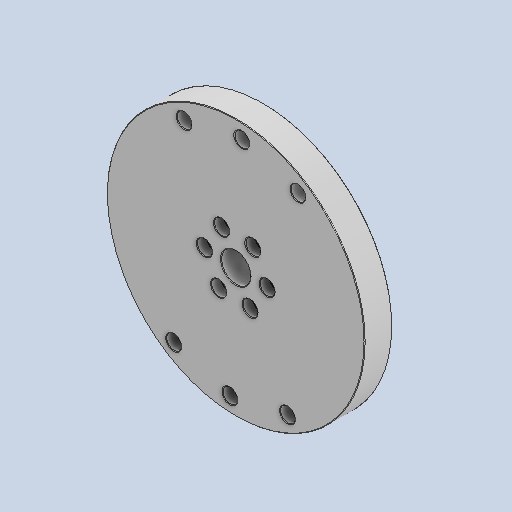
# Autodesk Inventor part: Góra
Saved by Autodesk Inventor 2023 (Build 270158000, 158)
## iProperties
Created: 2022-12-12
Part Number: Góra
Material: Generic
Document SubType Name: Modeling
Designer: komputer
Density: 1 g/cm^3
Appearance: Default
Author: komputer
Autodesk Inventor part; units mm, degrees
ref_plane "YZ Plane" through (0, 0, 0) normal (1, 0, 0) x (0, 1, 0)
ref_plane "XZ Plane" through (0, 0, 0) normal (0, 1, 0) x (-1, 0, 0)
ref_plane "XY Plane" through (0, 0, 0) normal (0, 0, 1) x (1, 0, 0)
sketch "Sketch1" plane through (0, 0, 0) normal (0, 0, 1) x (1, 0, 0)
  circle A0 centre (-9.0642, 40.3091) radius 2 projected
  circle A1 centre (-10.6114, 10.7871) radius 2 projected
  circle A2 centre (15.729, 24.2082) radius 2 projected
  circle A3 centre (6.4332, 9.8938) radius 2 projected
  circle A4 centre (-18.3601, 25.9947) radius 2 projected
  circle A5 centre (7.9804, 39.4158) radius 2 projected
  circle A6 centre (-1.3155, 25.1014) radius 9 projected
  circle A7 centre (-1.3155, 25.1014) radius 24.1359 projected
  circle A8 centre (-1.3155, 25.1014) radius 25 projected
  circle A9 centre (-9.0642, 40.3091) radius 3.5 projected
  circle A10 centre (-10.6114, 10.7871) radius 3.5 projected
  circle A11 centre (15.729, 24.2082) radius 3.5 projected
  circle A12 centre (6.4332, 9.8938) radius 3.5 projected
  circle A13 centre (-18.3601, 25.9947) radius 3.5 projected
  circle A14 centre (7.9804, 39.4158) radius 3.5 projected
  arc A15 (-0.8701, 59.0939) -> (-1.7609, 59.0939) centre (-1.3155, 25.1014) ccw projected
  arc A16 (1.7947, 58.9543) -> (-0.8701, 59.0939) centre (-1.3155, 25.1014) ccw projected
  arc A17 (2.6806, 58.8612) -> (1.7947, 58.9543) centre (-1.3155, 25.1014) ccw projected
  arc A18 (5.3163, 58.4437) -> (2.6806, 58.8612) centre (-1.3155, 25.1014) ccw projected
  arc A19 (6.1876, 58.2585) -> (5.3163, 58.4437) centre (-1.3155, 25.1014) ccw projected
  arc A20 (8.7652, 57.5678) -> (6.1876, 58.2585) centre (-1.3155, 25.1014) ccw projected
  arc A21 (9.6123, 57.2926) -> (8.7652, 57.5678) centre (-1.3155, 25.1014) ccw projected
  arc A22 (12.1036, 56.3363) -> (9.6123, 57.2926) centre (-1.3155, 25.1014) ccw projected
  arc A23 (12.9173, 55.974) -> (12.1036, 56.3363) centre (-1.3155, 25.1014) ccw projected
  arc A24 (15.295, 54.7625) -> (12.9173, 55.974) centre (-1.3155, 25.1014) ccw projected
  arc A25 (16.0664, 54.3171) -> (15.295, 54.7625) centre (-1.3155, 25.1014) ccw projected
  arc A26 (18.3044, 52.8637) -> (16.0664, 54.3171) centre (-1.3155, 25.1014) ccw projected
  arc A27 (19.0251, 52.3401) -> (18.3044, 52.8637) centre (-1.3155, 25.1014) ccw projected
  arc A28 (21.0989, 50.6608) -> (19.0251, 52.3401) centre (-1.3155, 25.1014) ccw projected
  arc A29 (21.7609, 50.0648) -> (21.0989, 50.6608) centre (-1.3155, 25.1014) ccw projected
  arc A30 (23.6478, 48.1778) -> (21.7609, 50.0648) centre (-1.3155, 25.1014) ccw projected
  arc A31 (24.2438, 47.5159) -> (23.6478, 48.1778) centre (-1.3155, 25.1014) ccw projected
  arc A32 (25.9232, 45.442) -> (24.2438, 47.5159) centre (-1.3155, 25.1014) ccw projected
  arc A33 (26.4468, 44.7214) -> (25.9232, 45.442) centre (-1.3155, 25.1014) ccw projected
  arc A34 (27.9002, 42.4834) -> (26.4468, 44.7214) centre (-1.3155, 25.1014) ccw projected
  arc A35 (28.3455, 41.712) -> (27.9002, 42.4834) centre (-1.3155, 25.1014) ccw projected
  arc A36 (29.557, 39.3343) -> (28.3455, 41.712) centre (-1.3155, 25.1014) ccw projected
  arc A37 (29.9193, 38.5206) -> (29.557, 39.3343) centre (-1.3155, 25.1014) ccw projected
  arc A38 (30.8756, 36.0293) -> (29.9193, 38.5206) centre (-1.3155, 25.1014) ccw projected
  arc A39 (31.1509, 35.1821) -> (30.8756, 36.0293) centre (-1.3155, 25.1014) ccw projected
  arc A40 (31.8416, 32.6045) -> (31.1509, 35.1821) centre (-1.3155, 25.1014) ccw projected
  arc A41 (32.0268, 31.7332) -> (31.8416, 32.6045) centre (-1.3155, 25.1014) ccw projected
  arc A42 (32.4442, 29.0976) -> (32.0268, 31.7332) centre (-1.3155, 25.1014) ccw projected
  arc A43 (32.5373, 28.2117) -> (32.4442, 29.0976) centre (-1.3155, 25.1014) ccw projected
  arc A44 (32.677, 25.5468) -> (32.5373, 28.2117) centre (-1.3155, 25.1014) ccw projected
  arc A45 (32.677, 24.6561) -> (32.677, 25.5468) centre (-1.3155, 25.1014) ccw projected
  arc A46 (32.5373, 21.9912) -> (32.677, 24.6561) centre (-1.3155, 25.1014) ccw projected
  arc A47 (32.4442, 21.1053) -> (32.5373, 21.9912) centre (-1.3155, 25.1014) ccw projected
  arc A48 (32.0268, 18.4697) -> (32.4442, 21.1053) centre (-1.3155, 25.1014) ccw projected
  arc A49 (31.8416, 17.5984) -> (32.0268, 18.4697) centre (-1.3155, 25.1014) ccw projected
  arc A50 (31.1509, 15.0208) -> (31.8416, 17.5984) centre (-1.3155, 25.1014) ccw projected
  arc A51 (30.8756, 14.1736) -> (31.1509, 15.0208) centre (-1.3155, 25.1014) ccw projected
  arc A52 (29.9193, 11.6823) -> (30.8756, 14.1736) centre (-1.3155, 25.1014) ccw projected
  arc A53 (29.557, 10.8686) -> (29.9193, 11.6823) centre (-1.3155, 25.1014) ccw projected
  arc A54 (28.3455, 8.4909) -> (29.557, 10.8686) centre (-1.3155, 25.1014) ccw projected
  arc A55 (27.9002, 7.7195) -> (28.3455, 8.4909) centre (-1.3155, 25.1014) ccw projected
  arc A56 (26.4468, 5.4815) -> (27.9002, 7.7195) centre (-1.3155, 25.1014) ccw projected
  arc A57 (25.9232, 4.7608) -> (26.4468, 5.4815) centre (-1.3155, 25.1014) ccw projected
  arc A58 (24.2438, 2.687) -> (25.9232, 4.7608) centre (-1.3155, 25.1014) ccw projected
  arc A59 (23.6478, 2.0251) -> (24.2438, 2.687) centre (-1.3155, 25.1014) ccw projected
  arc A60 (21.7609, 0.1381) -> (23.6478, 2.0251) centre (-1.3155, 25.1014) ccw projected
  arc A61 (21.0989, -0.4579) -> (21.7609, 0.1381) centre (-1.3155, 25.1014) ccw projected
  arc A62 (19.0251, -2.1373) -> (21.0989, -0.4579) centre (-1.3155, 25.1014) ccw projected
  arc A63 (18.3044, -2.6608) -> (19.0251, -2.1373) centre (-1.3155, 25.1014) ccw projected
  arc A64 (16.0664, -4.1142) -> (18.3044, -2.6608) centre (-1.3155, 25.1014) ccw projected
  arc A65 (15.295, -4.5596) -> (16.0664, -4.1142) centre (-1.3155, 25.1014) ccw projected
  arc A66 (12.9173, -5.7711) -> (15.295, -4.5596) centre (-1.3155, 25.1014) ccw projected
  arc A67 (12.1036, -6.1334) -> (12.9173, -5.7711) centre (-1.3155, 25.1014) ccw projected
  arc A68 (9.6123, -7.0897) -> (12.1036, -6.1334) centre (-1.3155, 25.1014) ccw projected
  arc A69 (8.7652, -7.365) -> (9.6123, -7.0897) centre (-1.3155, 25.1014) ccw projected
  arc A70 (6.1876, -8.0556) -> (8.7652, -7.365) centre (-1.3155, 25.1014) ccw projected
  arc A71 (5.3163, -8.2408) -> (6.1876, -8.0556) centre (-1.3155, 25.1014) ccw projected
  arc A72 (2.6806, -8.6583) -> (5.3163, -8.2408) centre (-1.3155, 25.1014) ccw projected
  arc A73 (1.7947, -8.7514) -> (2.6806, -8.6583) centre (-1.3155, 25.1014) ccw projected
  arc A74 (-0.8701, -8.891) -> (1.7947, -8.7514) centre (-1.3155, 25.1014) ccw projected
  arc A75 (-1.7609, -8.891) -> (-0.8701, -8.891) centre (-1.3155, 25.1014) ccw projected
  arc A76 (-4.4258, -8.7514) -> (-1.7609, -8.891) centre (-1.3155, 25.1014) ccw projected
  arc A77 (-5.3116, -8.6583) -> (-4.4258, -8.7514) centre (-1.3155, 25.1014) ccw projected
  arc A78 (-7.9473, -8.2408) -> (-5.3116, -8.6583) centre (-1.3155, 25.1014) ccw projected
  arc A79 (-8.8186, -8.0556) -> (-7.9473, -8.2408) centre (-1.3155, 25.1014) ccw projected
  arc A80 (-11.3962, -7.365) -> (-8.8186, -8.0556) centre (-1.3155, 25.1014) ccw projected
  arc A81 (-12.2433, -7.0897) -> (-11.3962, -7.365) centre (-1.3155, 25.1014) ccw projected
  arc A82 (-14.7346, -6.1334) -> (-12.2433, -7.0897) centre (-1.3155, 25.1014) ccw projected
  arc A83 (-15.5484, -5.7711) -> (-14.7346, -6.1334) centre (-1.3155, 25.1014) ccw projected
  arc A84 (-17.926, -4.5596) -> (-15.5484, -5.7711) centre (-1.3155, 25.1014) ccw projected
  arc A85 (-18.6975, -4.1142) -> (-17.926, -4.5596) centre (-1.3155, 25.1014) ccw projected
  arc A86 (-20.9355, -2.6608) -> (-18.6975, -4.1142) centre (-1.3155, 25.1014) ccw projected
  arc A87 (-21.6561, -2.1373) -> (-20.9355, -2.6608) centre (-1.3155, 25.1014) ccw projected
  arc A88 (-23.7299, -0.4579) -> (-21.6561, -2.1373) centre (-1.3155, 25.1014) ccw projected
  arc A89 (-24.3919, 0.1381) -> (-23.7299, -0.4579) centre (-1.3155, 25.1014) ccw projected
  arc A90 (-26.2788, 2.0251) -> (-24.3919, 0.1381) centre (-1.3155, 25.1014) ccw projected
  arc A91 (-26.8749, 2.687) -> (-26.2788, 2.0251) centre (-1.3155, 25.1014) ccw projected
  arc A92 (-28.5542, 4.7608) -> (-26.8749, 2.687) centre (-1.3155, 25.1014) ccw projected
  arc A93 (-29.0778, 5.4815) -> (-28.5542, 4.7608) centre (-1.3155, 25.1014) ccw projected
  arc A94 (-30.5312, 7.7195) -> (-29.0778, 5.4815) centre (-1.3155, 25.1014) ccw projected
  arc A95 (-30.9766, 8.4909) -> (-30.5312, 7.7195) centre (-1.3155, 25.1014) ccw projected
  arc A96 (-32.188, 10.8686) -> (-30.9766, 8.4909) centre (-1.3155, 25.1014) ccw projected
  arc A97 (-32.5503, 11.6823) -> (-32.188, 10.8686) centre (-1.3155, 25.1014) ccw projected
  arc A98 (-33.5067, 14.1736) -> (-32.5503, 11.6823) centre (-1.3155, 25.1014) ccw projected
  arc A99 (-33.7819, 15.0208) -> (-33.5067, 14.1736) centre (-1.3155, 25.1014) ccw projected
  arc A100 (-34.4726, 17.5984) -> (-33.7819, 15.0208) centre (-1.3155, 25.1014) ccw projected
  arc A101 (-34.6578, 18.4697) -> (-34.4726, 17.5984) centre (-1.3155, 25.1014) ccw projected
  arc A102 (-35.0752, 21.1053) -> (-34.6578, 18.4697) centre (-1.3155, 25.1014) ccw projected
  arc A103 (-35.1683, 21.9912) -> (-35.0752, 21.1053) centre (-1.3155, 25.1014) ccw projected
  arc A104 (-35.308, 24.6561) -> (-35.1683, 21.9912) centre (-1.3155, 25.1014) ccw projected
  arc A105 (-35.308, 25.5468) -> (-35.308, 24.6561) centre (-1.3155, 25.1014) ccw projected
  arc A106 (-35.1683, 28.2117) -> (-35.308, 25.5468) centre (-1.3155, 25.1014) ccw projected
  arc A107 (-35.0752, 29.0976) -> (-35.1683, 28.2117) centre (-1.3155, 25.1014) ccw projected
  arc A108 (-34.6578, 31.7332) -> (-35.0752, 29.0976) centre (-1.3155, 25.1014) ccw projected
  arc A109 (-34.4726, 32.6045) -> (-34.6578, 31.7332) centre (-1.3155, 25.1014) ccw projected
  arc A110 (-33.7819, 35.1821) -> (-34.4726, 32.6045) centre (-1.3155, 25.1014) ccw projected
  arc A111 (-33.5067, 36.0293) -> (-33.7819, 35.1821) centre (-1.3155, 25.1014) ccw projected
  arc A112 (-32.5503, 38.5206) -> (-33.5067, 36.0293) centre (-1.3155, 25.1014) ccw projected
  arc A113 (-32.188, 39.3343) -> (-32.5503, 38.5206) centre (-1.3155, 25.1014) ccw projected
  arc A114 (-30.9766, 41.712) -> (-32.188, 39.3343) centre (-1.3155, 25.1014) ccw projected
  arc A115 (-30.5312, 42.4834) -> (-30.9766, 41.712) centre (-1.3155, 25.1014) ccw projected
  arc A116 (-29.0778, 44.7214) -> (-30.5312, 42.4834) centre (-1.3155, 25.1014) ccw projected
  arc A117 (-28.5542, 45.442) -> (-29.0778, 44.7214) centre (-1.3155, 25.1014) ccw projected
  arc A118 (-26.8749, 47.5159) -> (-28.5542, 45.442) centre (-1.3155, 25.1014) ccw projected
  arc A119 (-26.2788, 48.1778) -> (-26.8749, 47.5159) centre (-1.3155, 25.1014) ccw projected
  arc A120 (-24.3919, 50.0648) -> (-26.2788, 48.1778) centre (-1.3155, 25.1014) ccw projected
  arc A121 (-23.7299, 50.6608) -> (-24.3919, 50.0648) centre (-1.3155, 25.1014) ccw projected
  arc A122 (-21.6561, 52.3401) -> (-23.7299, 50.6608) centre (-1.3155, 25.1014) ccw projected
  arc A123 (-20.9355, 52.8637) -> (-21.6561, 52.3401) centre (-1.3155, 25.1014) ccw projected
  arc A124 (-18.6975, 54.3171) -> (-20.9355, 52.8637) centre (-1.3155, 25.1014) ccw projected
  arc A125 (-17.926, 54.7625) -> (-18.6975, 54.3171) centre (-1.3155, 25.1014) ccw projected
  arc A126 (-15.5484, 55.974) -> (-17.926, 54.7625) centre (-1.3155, 25.1014) ccw projected
  arc A127 (-14.7346, 56.3363) -> (-15.5484, 55.974) centre (-1.3155, 25.1014) ccw projected
  arc A128 (-12.2433, 57.2926) -> (-14.7346, 56.3363) centre (-1.3155, 25.1014) ccw projected
  arc A129 (-11.3962, 57.5678) -> (-12.2433, 57.2926) centre (-1.3155, 25.1014) ccw projected
  arc A130 (-8.8186, 58.2585) -> (-11.3962, 57.5678) centre (-1.3155, 25.1014) ccw projected
  arc A131 (-7.9473, 58.4437) -> (-8.8186, 58.2585) centre (-1.3155, 25.1014) ccw projected
  arc A132 (-5.3116, 58.8612) -> (-7.9473, 58.4437) centre (-1.3155, 25.1014) ccw projected
  arc A133 (-4.4258, 58.9543) -> (-5.3116, 58.8612) centre (-1.3155, 25.1014) ccw projected
  arc A134 (-1.7609, 59.0939) -> (-4.4258, 58.9543) centre (-1.3155, 25.1014) ccw projected
  circle A135 centre (-1.3155, 25.1014) radius 9 projected
  circle A136 centre (-1.3155, 25.1014) radius 8 projected
  point P0 (0, 0)
extrude "Extrusion1" add sketch "Sketch1" along normal blind 37 contours A6 | A7 | A9 | A10 | A11 | A12 | A13 | A14
sketch "Sketch2" plane through (-1.3155, 25.1014, 37) normal (0, 0, 1) x (1, 0, 0)
  circle A0 centre (0, 0) radius 43.6804 projected
  circle A1 centre (0, 0) radius 8 projected
  circle A2 centre (0, 0) radius 50
  circle A3 centre (0, 0) radius 24.1359 projected
  circle A4 centre (9.2959, 14.3144) radius 2 projected
  circle A5 centre (-17.0446, 0.8933) radius 2 projected
  circle A6 centre (7.7487, -15.2076) radius 2 projected
  circle A7 centre (17.0446, -0.8933) radius 2 projected
  circle A8 centre (-9.2959, -14.3144) radius 2 projected
  circle A9 centre (-7.7487, 15.2076) radius 2 projected
  circle A10 centre (0, 0) radius 8 projected
  point P0 (1.3155, -25.1014)
  dimension "d2" = 100
  constraints: 1 centre point, 1 coincident
  measures "d2" diameter of A2
extrude "Extrusion2" add sketch "Sketch2" against normal blind 10 contours A0 | A2
sketch "Sketch3" plane through (-1.3155, 25.1014, 37) normal (0, 0, 1) x (1, 0, 0)
  circle A0 centre (0, 0) radius 55
  circle A1 centre (0, 0) radius 50 projected
  circle A2 centre (9.2959, 14.3144) radius 2 projected
  circle A3 centre (-17.0446, 0.8933) radius 2 projected
  circle A4 centre (7.7487, -15.2076) radius 2 projected
  circle A5 centre (17.0446, -0.8933) radius 2 projected
  circle A6 centre (-9.2959, -14.3144) radius 2 projected
  circle A7 centre (-7.7487, 15.2076) radius 2 projected
  circle A8 centre (0, 0) radius 8 projected
  point P0 (1.3155, -25.1014)
  constraints: 1 centre point, 2 other
ref_plane "Work Plane1" through (-65.2569, -38.84, 26) normal (0, 0, 1) x (0.9839108, 0.1786605, 0)
extrude "Extrusion3" add sketch "Sketch3" against normal blind 10 contours A0
sketch "Sketch4" plane through (-1.3155, 25.1014, 37) normal (0, 0, 1) x (1, 0, 0)
  circle A0 centre (0, 0) radius 55 projected
  circle A1 centre (9.2959, 14.3144) radius 2 projected
  circle A2 centre (-17.0446, 0.8933) radius 2 projected
  circle A3 centre (7.7487, -15.2076) radius 2 projected
  circle A4 centre (17.0446, -0.8933) radius 2 projected
  circle A5 centre (-9.2959, -14.3144) radius 2 projected
  circle A6 centre (-7.7487, 15.2076) radius 2 projected
  circle A7 centre (0, 0) radius 8 projected
  line L0 (-9.2959, -14.3144) -> (-9.2959, -10.8144)
  line L1 (-9.2959, -10.8144) -> (-9.2959, -17.4144)
  line L2 (-11.0857, -17.4144) -> (-12.8754, -14.3144)
  line L3 (-12.8754, -14.3144) -> (-11.0857, -11.2144)
  line L4 (-11.0857, -11.2144) -> (-7.5061, -11.2144)
  line L5 (-7.5061, -11.2144) -> (-5.7163, -14.3144)
  line L6 (-5.7163, -14.3144) -> (-7.5061, -17.4144)
  line L7 (-7.5061, -17.4144) -> (-11.0857, -17.4144)
  line L8 (9.5385, -12.1076) -> (11.3283, -15.2076)
  line L9 (9.5385, -18.3076) -> (5.9589, -18.3076)
  line L10 (5.9589, -18.3076) -> (4.1691, -15.2076)
  line L11 (11.3283, -15.2076) -> (9.5385, -18.3076)
  line L12 (4.1691, -15.2076) -> (5.9589, -12.1076)
  line L13 (5.9589, -12.1076) -> (9.5385, -12.1076)
  line L14 (15.2548, 2.2067) -> (18.8343, 2.2067)
  line L15 (20.6241, -0.8933) -> (18.8343, -3.9933)
  line L16 (18.8343, -3.9933) -> (15.2548, -3.9933)
  line L17 (18.8343, 2.2067) -> (20.6241, -0.8933)
  line L18 (15.2548, -3.9933) -> (13.465, -0.8933)
  line L19 (13.465, -0.8933) -> (15.2548, 2.2067)
  line L20 (5.7163, 14.3144) -> (7.5061, 17.4144)
  line L21 (11.0857, 17.4144) -> (12.8754, 14.3144)
  line L22 (12.8754, 14.3144) -> (11.0857, 11.2144)
  line L23 (7.5061, 17.4144) -> (11.0857, 17.4144)
  line L24 (11.0857, 11.2144) -> (7.5061, 11.2144)
  line L25 (7.5061, 11.2144) -> (5.7163, 14.3144)
  line L26 (-9.5385, 12.1076) -> (-11.3283, 15.2076)
  line L27 (-9.5385, 18.3076) -> (-5.9589, 18.3076)
  line L28 (-5.9589, 18.3076) -> (-4.1691, 15.2076)
  line L29 (-11.3283, 15.2076) -> (-9.5385, 18.3076)
  line L30 (-4.1691, 15.2076) -> (-5.9589, 12.1076)
  line L31 (-5.9589, 12.1076) -> (-9.5385, 12.1076)
  line L32 (-15.2548, -2.2067) -> (-18.8343, -2.2067)
  line L33 (-20.6241, 0.8933) -> (-18.8343, 3.9933)
  line L34 (-18.8343, 3.9933) -> (-15.2548, 3.9933)
  line L35 (-18.8343, -2.2067) -> (-20.6241, 0.8933)
  line L36 (-15.2548, 3.9933) -> (-13.465, 0.8933)
  line L37 (-13.465, 0.8933) -> (-15.2548, -2.2067)
  point P0 (1.3155, -25.1014)
  point P1 (10.4334, -16.7576)
  point P2 (7.7487, -15.2076)
  point P3 (4.7176, -13.4576)
  point P4 (19.7292, 0.6567)
  point P5 (17.0446, -0.8933)
  point P6 (14.0135, -2.6433)
  point P7 (9.2959, 17.4144)
  point P8 (9.2959, 14.3144)
  point P9 (9.2959, 10.8144)
  point P10 (-10.4334, 16.7576)
  point P11 (-7.7487, 15.2076)
  point P12 (-4.7176, 13.4576)
  point P13 (-19.7292, -0.6567)
  point P14 (-17.0446, 0.8933)
  point P15 (-14.0135, 2.6433)
  dimension "d7" = 3.5
  dimension "d8" = 6.6
  dimension "d11" = 360
  constraints: 76 end point, 2 coincident, 1 midpoint, 1 point on line, 1 vertical, 104 other
  measures "d7" distance of L0.start L0.end
  measures "d8" distance of L0.end L1.end
extrude "Extrusion4" cut sketch "Sketch4" against normal blind 5.4 contours A1 | A2 | A3 | A4 | A5 L1 L0 | A5 L0 L4 L5 L6 L7 L1 | L0 L1 A5 | A5 L1 L7 L2 L3 L4 L0 | A6 | L8 L11 L9 L10 L12 L13 | L14 L17 L15 L16 L18 L19 | L20 L23 L21 L22 L24 L25 | L26 L29 L27 L28 L30 L31 | L32 L35 L33 L34 L36 L37
sketch "Sketch14" plane through (-1.3155, 25.1014, 37) normal (0, 0, 1) x (1, 0, 0)
  circle A0 centre (0, 0) radius 55 projected
  line L0 (-7.5061, -11.2144) -> (-5.7163, -14.3144) projected
  line L1 (-5.7163, -14.3144) -> (-7.5061, -17.4144) projected
  line L2 (-7.5061, -17.4144) -> (-11.0857, -17.4144) projected
  line L3 (-11.0857, -17.4144) -> (-12.8754, -14.3144) projected
  line L4 (-12.8754, -14.3144) -> (-11.0857, -11.2144) projected
  line L5 (-11.0857, -11.2144) -> (-7.5061, -11.2144) projected
  line L6 (18.8343, -3.9933) -> (15.2548, -3.9933) projected
  line L7 (15.2548, -3.9933) -> (13.465, -0.8933) projected
  line L8 (13.465, -0.8933) -> (15.2548, 2.2067) projected
  line L9 (15.2548, 2.2067) -> (18.8343, 2.2067) projected
  line L10 (18.8343, 2.2067) -> (20.6241, -0.8933) projected
  line L11 (20.6241, -0.8933) -> (18.8343, -3.9933) projected
  line L12 (12.8754, 14.3144) -> (11.0857, 11.2144) projected
  line L13 (11.0857, 11.2144) -> (7.5061, 11.2144) projected
  line L14 (7.5061, 11.2144) -> (5.7163, 14.3144) projected
  line L15 (5.7163, 14.3144) -> (7.5061, 17.4144) projected
  line L16 (7.5061, 17.4144) -> (11.0857, 17.4144) projected
  line L17 (11.0857, 17.4144) -> (12.8754, 14.3144) projected
  line L18 (-18.8343, 3.9933) -> (-15.2548, 3.9933) projected
  line L19 (-15.2548, 3.9933) -> (-13.465, 0.8933) projected
  line L20 (-13.465, 0.8933) -> (-15.2548, -2.2067) projected
  line L21 (-15.2548, -2.2067) -> (-18.8343, -2.2067) projected
  line L22 (-18.8343, -2.2067) -> (-20.6241, 0.8933) projected
  line L23 (-20.6241, 0.8933) -> (-18.8343, 3.9933) projected
  line L24 (5.9589, -18.3076) -> (4.1691, -15.2076) projected
  line L25 (4.1691, -15.2076) -> (5.9589, -12.1076) projected
  line L26 (5.9589, -12.1076) -> (9.5385, -12.1076) projected
  line L27 (9.5385, -12.1076) -> (11.3283, -15.2076) projected
  line L28 (11.3283, -15.2076) -> (9.5385, -18.3076) projected
  line L29 (9.5385, -18.3076) -> (5.9589, -18.3076) projected
  line L30 (-5.9589, 18.3076) -> (-4.1691, 15.2076) projected
  line L31 (-4.1691, 15.2076) -> (-5.9589, 12.1076) projected
  line L32 (-5.9589, 12.1076) -> (-9.5385, 12.1076) projected
  line L33 (-9.5385, 12.1076) -> (-11.3283, 15.2076) projected
  line L34 (-11.3283, 15.2076) -> (-9.5385, 18.3076) projected
  line L35 (-9.5385, 18.3076) -> (-5.9589, 18.3076) projected
  circle A1 centre (-9.2959, -14.3144) radius 2 projected
  circle A2 centre (7.7487, -15.2076) radius 2 projected
  circle A3 centre (9.2959, 14.3144) radius 2 projected
  circle A4 centre (-7.7487, 15.2076) radius 2 projected
  circle A5 centre (7.7487, -15.2076) radius 2 projected
  line L36 (-9.2959, -14.3144) -> (7.7487, -15.2076)
  line L37 (-7.7487, 15.2076) -> (9.2959, 14.3144)
  line L38 (0, 0) -> (-0.7736, -14.761)
  line L39 (0, 0) -> (0.7736, 14.761)
  line L40 (0, 0) -> (2.3551, 44.9383)
  circle A6 centre (0, 0) radius 8 projected
  line L41 (0, 0) -> (-2.3551, -44.9383)
  line L42 (-2.3551, -44.9383) -> (-54.5095, -42.205)
  line L43 (-54.5095, -42.205) -> (48.6276, -47.6102)
  line L44 (2.3551, 44.9383) -> (-54.5095, 47.9185)
  line L45 (2.3551, 44.9383) -> (72.9393, 41.2392)
  line L46 (2.3551, 44.9383) -> (3.5065, 66.9082)
  line L47 (0, 0) -> (-7.7487, 15.2076)
  line L48 (-7.7487, 15.2076) -> (-23.59, 46.2981)
  line L49 (-23.59, 46.2981) -> (-32.6698, 64.1182)
  circle A7 centre (0, 0) radius 71.9615
  circle A8 centre (-28.1299, 55.2081) radius 4
  circle A9 centre (-51.9653, 33.7467) radius 4
  circle A10 centre (-61.8766, 3.2428) radius 4
  circle A11 centre (-55.2081, -28.1299) radius 4
  circle A12 centre (-33.7467, -51.9653) radius 4
  circle A13 centre (-3.2428, -61.8766) radius 4
  circle A14 centre (28.1299, -55.2081) radius 4
  circle A15 centre (51.9653, -33.7467) radius 4
  circle A16 centre (61.8766, -3.2428) radius 4
  circle A17 centre (55.2081, 28.1299) radius 4
  circle A18 centre (33.7467, 51.9653) radius 4
  circle A19 centre (3.2428, 61.8766) radius 4
  line L50 (-2.3551, -44.9383) -> (-68.6558, -41.4637)
  line L51 (-68.6558, -41.4637) -> (71.9615, -48.8331)
  point P0 (1.3155, -25.1014)
  dimension "d60" = 45
  dimension "d61" = 45
  dimension "d62" = 22
  dimension "d63" = 20
  dimension "d65" = 8
  dimension "d69" = 360
  constraints: 32 end point, 12 centre point, 3 collinear, 3 midpoint, 3 perpendicular, 3 point on line, 2 coincident, 28 other
  measures "d60" distance of L38.start L40.end
  measures "d61" distance of L41.start L41.end
  measures "d62" distance of L40.end L46.end
  measures "d63" distance of L48.end L49.end
  measures "d65" diameter of A8
extrude "Extrusion16" add sketch "Sketch14" against normal up to surface (10 mm away) contours A0 L45 A7 L51 L43 | A0 L49 A8 A7 L45 | L43 L51 A7 L50 L42 A0 | L42 L50 A7 L44 A0 | A0 L44 A7 L49 A8 | A9 | A10 | A11 | A15 | A16 | A17
sketch "Sketch15" plane through (-1.3155, 25.1014, 37) normal (0, 0, 1) x (1, 0, 0)
  circle A0 centre (-28.1299, 55.2081) radius 4 projected
  circle A1 centre (33.7467, 51.9653) radius 4 projected
  circle A2 centre (-33.7467, -51.9653) radius 4 projected
  circle A3 centre (-3.2428, -61.8766) radius 4 projected
  circle A4 centre (28.1299, -55.2081) radius 4 projected
  circle A5 centre (3.2428, 61.8766) radius 4 projected
  circle A6 centre (0, 0) radius 71.9615 projected
  line L0 (-7.5061, -11.2144) -> (-5.7163, -14.3144) projected
  line L1 (-5.7163, -14.3144) -> (-7.5061, -17.4144) projected
  line L2 (-7.5061, -17.4144) -> (-11.0857, -17.4144) projected
  line L3 (-11.0857, -17.4144) -> (-12.8754, -14.3144) projected
  line L4 (-12.8754, -14.3144) -> (-11.0857, -11.2144) projected
  line L5 (-11.0857, -11.2144) -> (-7.5061, -11.2144) projected
  line L6 (18.8343, -3.9933) -> (15.2548, -3.9933) projected
  line L7 (15.2548, -3.9933) -> (13.465, -0.8933) projected
  line L8 (13.465, -0.8933) -> (15.2548, 2.2067) projected
  line L9 (15.2548, 2.2067) -> (18.8343, 2.2067) projected
  line L10 (18.8343, 2.2067) -> (20.6241, -0.8933) projected
  line L11 (20.6241, -0.8933) -> (18.8343, -3.9933) projected
  line L12 (12.8754, 14.3144) -> (11.0857, 11.2144) projected
  line L13 (11.0857, 11.2144) -> (7.5061, 11.2144) projected
  line L14 (7.5061, 11.2144) -> (5.7163, 14.3144) projected
  line L15 (5.7163, 14.3144) -> (7.5061, 17.4144) projected
  line L16 (7.5061, 17.4144) -> (11.0857, 17.4144) projected
  line L17 (11.0857, 17.4144) -> (12.8754, 14.3144) projected
  line L18 (-18.8343, 3.9933) -> (-15.2548, 3.9933) projected
  line L19 (-15.2548, 3.9933) -> (-13.465, 0.8933) projected
  line L20 (-13.465, 0.8933) -> (-15.2548, -2.2067) projected
  line L21 (-15.2548, -2.2067) -> (-18.8343, -2.2067) projected
  line L22 (-18.8343, -2.2067) -> (-20.6241, 0.8933) projected
  line L23 (-20.6241, 0.8933) -> (-18.8343, 3.9933) projected
  line L24 (5.9589, -18.3076) -> (4.1691, -15.2076) projected
  line L25 (4.1691, -15.2076) -> (5.9589, -12.1076) projected
  line L26 (5.9589, -12.1076) -> (9.5385, -12.1076) projected
  line L27 (9.5385, -12.1076) -> (11.3283, -15.2076) projected
  line L28 (11.3283, -15.2076) -> (9.5385, -18.3076) projected
  line L29 (9.5385, -18.3076) -> (5.9589, -18.3076) projected
  line L30 (-5.9589, 18.3076) -> (-4.1691, 15.2076) projected
  line L31 (-4.1691, 15.2076) -> (-5.9589, 12.1076) projected
  line L32 (-5.9589, 12.1076) -> (-9.5385, 12.1076) projected
  line L33 (-9.5385, 12.1076) -> (-11.3283, 15.2076) projected
  line L34 (-11.3283, 15.2076) -> (-9.5385, 18.3076) projected
  line L35 (-9.5385, 18.3076) -> (-5.9589, 18.3076) projected
  circle A7 centre (0, 0) radius 70
  point P0 (1.3155, -25.1014)
  dimension "d73" = 140
  constraints: 1 centre point
  measures "d73" diameter of A7
extrude "Extrusion17" cut sketch "Sketch15" against normal through all contours A6
sketch "Sketch16" plane through (-1.3155, 25.1014, 27) normal (0, 0, -1) x (-1, 0, 0)
  circle A0 centre (0, 0) radius 70 projected
  circle A1 centre (-3.2428, 61.8766) radius 4 projected
  circle A2 centre (-28.1299, -55.2081) radius 4 projected
  circle A3 centre (3.2428, -61.8766) radius 4 projected
  circle A4 centre (33.7467, -51.9653) radius 4 projected
  circle A5 centre (-33.7467, 51.9653) radius 4 projected
  circle A6 centre (28.1299, 55.2081) radius 4 projected
  circle A7 centre (0, 0) radius 24.1359 projected
  circle A8 centre (-28.1299, -55.2081) radius 4 projected
  circle A9 centre (28.1299, 55.2081) radius 4 projected
  line L0 (-28.1299, -55.2081) -> (28.1299, 55.2081)
  line L1 (-28.1299, -55.2081) -> (-25.3152, -49.6839)
  line L2 (-22.1258, -51.309) -> (-21.7511, -58.4583)
  line L3 (-21.7511, -58.4583) -> (-27.7553, -62.3575)
  line L4 (-27.7553, -62.3575) -> (-34.1341, -59.1073)
  line L5 (-34.1341, -59.1073) -> (-34.5088, -51.9579)
  line L6 (-34.5088, -51.9579) -> (-28.5046, -48.0588)
  line L7 (-28.5046, -48.0588) -> (-22.1258, -51.309)
  line L8 (-0.6563, -55.8724) -> (6.493, -55.4978)
  line L9 (-3.9065, -62.2513) -> (-0.6563, -55.8724)
  line L10 (-0.0074, -68.2555) -> (-3.9065, -62.2513)
  line L11 (7.142, -67.8808) -> (-0.0074, -68.2555)
  line L12 (10.3921, -61.5019) -> (7.142, -67.8808)
  line L13 (6.493, -55.4978) -> (10.3921, -61.5019)
  line L14 (27.3678, -48.7151) -> (33.372, -44.816)
  line L15 (27.7425, -55.8645) -> (27.3678, -48.7151)
  line L16 (34.1213, -59.1146) -> (27.7425, -55.8645)
  line L17 (40.1255, -55.2155) -> (34.1213, -59.1146)
  line L18 (39.7508, -48.0662) -> (40.1255, -55.2155)
  line L19 (33.372, -44.816) -> (39.7508, -48.0662)
  line L20 (48.0588, -28.5046) -> (51.309, -22.1258)
  line L21 (51.9579, -34.5088) -> (48.0588, -28.5046)
  line L22 (59.1073, -34.1341) -> (51.9579, -34.5088)
  line L23 (62.3575, -27.7553) -> (59.1073, -34.1341)
  line L24 (58.4583, -21.7511) -> (62.3575, -27.7553)
  line L25 (51.309, -22.1258) -> (58.4583, -21.7511)
  line L26 (55.8724, -0.6563) -> (55.4978, 6.493)
  line L27 (62.2513, -3.9065) -> (55.8724, -0.6563)
  line L28 (68.2555, -0.0074) -> (62.2513, -3.9065)
  line L29 (67.8808, 7.142) -> (68.2555, -0.0074)
  line L30 (61.5019, 10.3921) -> (67.8808, 7.142)
  line L31 (55.4978, 6.493) -> (61.5019, 10.3921)
  line L32 (48.7151, 27.3678) -> (44.816, 33.372)
  line L33 (55.8645, 27.7425) -> (48.7151, 27.3678)
  line L34 (59.1146, 34.1213) -> (55.8645, 27.7425)
  line L35 (55.2155, 40.1255) -> (59.1146, 34.1213)
  line L36 (48.0662, 39.7508) -> (55.2155, 40.1255)
  line L37 (44.816, 33.372) -> (48.0662, 39.7508)
  line L38 (28.5046, 48.0588) -> (22.1258, 51.309)
  line L39 (34.5088, 51.9579) -> (28.5046, 48.0588)
  line L40 (34.1341, 59.1073) -> (34.5088, 51.9579)
  line L41 (27.7553, 62.3575) -> (34.1341, 59.1073)
  line L42 (21.7511, 58.4583) -> (27.7553, 62.3575)
  line L43 (22.1258, 51.309) -> (21.7511, 58.4583)
  line L44 (0.6563, 55.8724) -> (-6.493, 55.4978)
  line L45 (3.9065, 62.2513) -> (0.6563, 55.8724)
  line L46 (0.0074, 68.2555) -> (3.9065, 62.2513)
  line L47 (-7.142, 67.8808) -> (0.0074, 68.2555)
  line L48 (-10.3921, 61.5019) -> (-7.142, 67.8808)
  line L49 (-6.493, 55.4978) -> (-10.3921, 61.5019)
  line L50 (-27.3678, 48.7151) -> (-33.372, 44.816)
  line L51 (-27.7425, 55.8645) -> (-27.3678, 48.7151)
  line L52 (-34.1213, 59.1146) -> (-27.7425, 55.8645)
  line L53 (-40.1255, 55.2155) -> (-34.1213, 59.1146)
  line L54 (-39.7508, 48.0662) -> (-40.1255, 55.2155)
  line L55 (-33.372, 44.816) -> (-39.7508, 48.0662)
  line L56 (-48.0588, 28.5046) -> (-51.309, 22.1258)
  line L57 (-51.9579, 34.5088) -> (-48.0588, 28.5046)
  line L58 (-59.1073, 34.1341) -> (-51.9579, 34.5088)
  line L59 (-62.3575, 27.7553) -> (-59.1073, 34.1341)
  line L60 (-58.4583, 21.7511) -> (-62.3575, 27.7553)
  line L61 (-51.309, 22.1258) -> (-58.4583, 21.7511)
  line L62 (-55.8724, 0.6563) -> (-55.4978, -6.493)
  line L63 (-62.2513, 3.9065) -> (-55.8724, 0.6563)
  line L64 (-68.2555, 0.0074) -> (-62.2513, 3.9065)
  line L65 (-67.8808, -7.142) -> (-68.2555, 0.0074)
  line L66 (-61.5019, -10.3921) -> (-67.8808, -7.142)
  line L67 (-55.4978, -6.493) -> (-61.5019, -10.3921)
  line L68 (-48.7151, -27.3678) -> (-44.816, -33.372)
  line L69 (-55.8645, -27.7425) -> (-48.7151, -27.3678)
  line L70 (-59.1146, -34.1213) -> (-55.8645, -27.7425)
  line L71 (-55.2155, -40.1255) -> (-59.1146, -34.1213)
  line L72 (-48.0662, -39.7508) -> (-55.2155, -40.1255)
  line L73 (-44.816, -33.372) -> (-48.0662, -39.7508)
  point P0 (-1.3155, -25.1014)
  point P1 (2.9183, -55.6851)
  point P2 (30.3699, -46.7655)
  point P3 (49.6839, -25.3152)
  point P4 (55.6851, 2.9183)
  point P5 (46.7655, 30.3699)
  point P6 (25.3152, 49.6839)
  point P7 (-2.9183, 55.6851)
  point P8 (-30.3699, 46.7655)
  point P9 (-49.6839, 25.3152)
  point P10 (-55.6851, -2.9183)
  point P11 (-46.7655, -30.3699)
  dimension "d76" = 6.2
  dimension "d79" = 360
  constraints: 148 end point, 1 coincident, 1 midpoint, 1 point on line, 170 other
  measures "d76" distance of L0.start L1.end
extrude "Extrusion18" cut sketch "Sketch16" against normal blind 9 contours A1 | A2 | A3 | A4 | A5 | A6 | L2 L3 L4 L5 L6 L7 | L8 L13 L12 L11 L10 L9 | L14 L19 L18 L17 L16 L15 | L38 L43 L42 L41 L40 L39 | L44 L49 L48 L47 L46 L45 | L50 L55 L54 L53 L52 L51
sketch "Sketch17" plane through (-1.3155, 25.1014, 37) normal (0, 0, 1) x (1, 0, 0)
  circle A0 centre (0, 0) radius 70 projected
  circle A1 centre (-28.1299, 55.2081) radius 4 projected
  circle A2 centre (33.7467, 51.9653) radius 4 projected
  circle A3 centre (-33.7467, -51.9653) radius 4 projected
  circle A4 centre (-3.2428, -61.8766) radius 4 projected
  circle A5 centre (28.1299, -55.2081) radius 4 projected
  circle A6 centre (3.2428, 61.8766) radius 4 projected
  line L0 (-5.9589, 18.3076) -> (-4.1691, 15.2076) projected
  line L1 (-4.1691, 15.2076) -> (-5.9589, 12.1076) projected
  line L2 (-5.9589, 12.1076) -> (-9.5385, 12.1076) projected
  line L3 (-9.5385, 12.1076) -> (-11.3283, 15.2076) projected
  line L4 (-11.3283, 15.2076) -> (-9.5385, 18.3076) projected
  line L5 (-9.5385, 18.3076) -> (-5.9589, 18.3076) projected
  line L6 (5.9589, -18.3076) -> (4.1691, -15.2076) projected
  line L7 (4.1691, -15.2076) -> (5.9589, -12.1076) projected
  line L8 (5.9589, -12.1076) -> (9.5385, -12.1076) projected
  line L9 (9.5385, -12.1076) -> (11.3283, -15.2076) projected
  line L10 (11.3283, -15.2076) -> (9.5385, -18.3076) projected
  line L11 (9.5385, -18.3076) -> (5.9589, -18.3076) projected
  line L12 (-18.8343, 3.9933) -> (-15.2548, 3.9933) projected
  line L13 (-15.2548, 3.9933) -> (-13.465, 0.8933) projected
  line L14 (-13.465, 0.8933) -> (-15.2548, -2.2067) projected
  line L15 (-15.2548, -2.2067) -> (-18.8343, -2.2067) projected
  line L16 (-18.8343, -2.2067) -> (-20.6241, 0.8933) projected
  line L17 (-20.6241, 0.8933) -> (-18.8343, 3.9933) projected
  line L18 (12.8754, 14.3144) -> (11.0857, 11.2144) projected
  line L19 (11.0857, 11.2144) -> (7.5061, 11.2144) projected
  line L20 (7.5061, 11.2144) -> (5.7163, 14.3144) projected
  line L21 (5.7163, 14.3144) -> (7.5061, 17.4144) projected
  line L22 (7.5061, 17.4144) -> (11.0857, 17.4144) projected
  line L23 (11.0857, 17.4144) -> (12.8754, 14.3144) projected
  line L24 (18.8343, -3.9933) -> (15.2548, -3.9933) projected
  line L25 (15.2548, -3.9933) -> (13.465, -0.8933) projected
  line L26 (13.465, -0.8933) -> (15.2548, 2.2067) projected
  line L27 (15.2548, 2.2067) -> (18.8343, 2.2067) projected
  line L28 (18.8343, 2.2067) -> (20.6241, -0.8933) projected
  line L29 (20.6241, -0.8933) -> (18.8343, -3.9933) projected
  line L30 (-7.5061, -11.2144) -> (-5.7163, -14.3144) projected
  line L31 (-5.7163, -14.3144) -> (-7.5061, -17.4144) projected
  line L32 (-7.5061, -17.4144) -> (-11.0857, -17.4144) projected
  line L33 (-11.0857, -17.4144) -> (-12.8754, -14.3144) projected
  line L34 (-12.8754, -14.3144) -> (-11.0857, -11.2144) projected
  line L35 (-11.0857, -11.2144) -> (-7.5061, -11.2144) projected
  circle A7 centre (0, 0) radius 8 projected
  point P0 (1.3155, -25.1014)
extrude "Extrusion19" add sketch "Sketch17" along normal blind 5
sketch "Sketch18" plane through (-1.3155, 25.1014, 0) normal (0, 0, -1) x (-1, 0, 0)
  circle A0 centre (0, 0) radius 24.1359 projected
  circle A1 centre (-9.2959, 14.3144) radius 2 projected
  circle A2 centre (17.0446, 0.8933) radius 2 projected
  circle A3 centre (-7.7487, -15.2076) radius 2 projected
  circle A4 centre (-17.0446, -0.8933) radius 2 projected
  circle A5 centre (9.2959, -14.3144) radius 2 projected
  circle A6 centre (7.7487, 15.2076) radius 2 projected
  circle A7 centre (0, 0) radius 8 projected
  point P0 (-1.3155, -25.1014)
extrude "Extrusion20" cut sketch "Sketch18" against normal blind 10
sketch "Sketch19" plane through (-1.3155, 25.1014, 10) normal (0, 0, -1) x (-1, 0, 0)
  circle A0 centre (0, 0) radius 24.1359 projected
  circle A1 centre (0, 0) radius 8 projected
  circle A2 centre (7.7487, 15.2076) radius 2 projected
  circle A3 centre (9.2959, -14.3144) radius 2 projected
  circle A4 centre (-17.0446, -0.8933) radius 2 projected
  circle A5 centre (-7.7487, -15.2076) radius 2 projected
  circle A6 centre (17.0446, 0.8933) radius 2 projected
  circle A7 centre (-9.2959, 14.3144) radius 2 projected
  point P0 (-1.3155, -25.1014)
extrude "Extrusion21" cut sketch "Sketch19" against normal blind 10
sketch "Sketch20" plane through (-1.3155, 25.1014, 20) normal (0, 0, -1) x (-1, 0, 0)
  circle A0 centre (0, 0) radius 24.1359 projected
  circle A1 centre (-9.2959, 14.3144) radius 2 projected
  circle A2 centre (17.0446, 0.8933) radius 2 projected
  circle A3 centre (-7.7487, -15.2076) radius 2 projected
  circle A4 centre (-17.0446, -0.8933) radius 2 projected
  circle A5 centre (9.2959, -14.3144) radius 2 projected
  circle A6 centre (7.7487, 15.2076) radius 2 projected
  circle A7 centre (0, 0) radius 8 projected
  circle A8 centre (0, 0) radius 24.95
  point P0 (-1.3155, -25.1014)
  dimension "d89" = 49.9
  constraints: 1 centre point, 1 coincident
  measures "d89" diameter of A8
extrude "Extrusion22" add sketch "Sketch20" against normal up to surface (7 mm away) contours A8
sketch "Sketch21" plane through (-1.3155, 25.1014, 42) normal (0, 0, 1) x (1, 0, 0)
  circle A0 centre (9.2959, 14.3144) radius 2 projected
  circle A1 centre (17.0446, -0.8933) radius 2 projected
  circle A2 centre (7.7487, -15.2076) radius 2 projected
  circle A3 centre (-9.2959, -14.3144) radius 2 projected
  circle A4 centre (-17.0446, 0.8933) radius 2 projected
  circle A5 centre (-7.7487, 15.2076) radius 2 projected
  circle A6 centre (0, 0) radius 70 projected
  circle A7 centre (0, 0) radius 8 projected
  line L0 (-7.5061, -11.2144) -> (-5.7163, -14.3144) projected
  line L1 (-5.7163, -14.3144) -> (-7.5061, -17.4144) projected
  line L2 (-7.5061, -17.4144) -> (-11.0857, -17.4144) projected
  line L3 (-11.0857, -17.4144) -> (-12.8754, -14.3144) projected
  line L4 (-12.8754, -14.3144) -> (-11.0857, -11.2144) projected
  line L5 (-11.0857, -11.2144) -> (-7.5061, -11.2144) projected
  line L6 (18.8343, -3.9933) -> (15.2548, -3.9933) projected
  line L7 (15.2548, -3.9933) -> (13.465, -0.8933) projected
  line L8 (13.465, -0.8933) -> (15.2548, 2.2067) projected
  line L9 (15.2548, 2.2067) -> (18.8343, 2.2067) projected
  line L10 (18.8343, 2.2067) -> (20.6241, -0.8933) projected
  line L11 (20.6241, -0.8933) -> (18.8343, -3.9933) projected
  line L12 (12.8754, 14.3144) -> (11.0857, 11.2144) projected
  line L13 (11.0857, 11.2144) -> (7.5061, 11.2144) projected
  line L14 (7.5061, 11.2144) -> (5.7163, 14.3144) projected
  line L15 (5.7163, 14.3144) -> (7.5061, 17.4144) projected
  line L16 (7.5061, 17.4144) -> (11.0857, 17.4144) projected
  line L17 (11.0857, 17.4144) -> (12.8754, 14.3144) projected
  line L18 (-18.8343, 3.9933) -> (-15.2548, 3.9933) projected
  line L19 (-15.2548, 3.9933) -> (-13.465, 0.8933) projected
  line L20 (-13.465, 0.8933) -> (-15.2548, -2.2067) projected
  line L21 (-15.2548, -2.2067) -> (-18.8343, -2.2067) projected
  line L22 (-18.8343, -2.2067) -> (-20.6241, 0.8933) projected
  line L23 (-20.6241, 0.8933) -> (-18.8343, 3.9933) projected
  line L24 (5.9589, -18.3076) -> (4.1691, -15.2076) projected
  line L25 (4.1691, -15.2076) -> (5.9589, -12.1076) projected
  line L26 (5.9589, -12.1076) -> (9.5385, -12.1076) projected
  line L27 (9.5385, -12.1076) -> (11.3283, -15.2076) projected
  line L28 (11.3283, -15.2076) -> (9.5385, -18.3076) projected
  line L29 (9.5385, -18.3076) -> (5.9589, -18.3076) projected
  line L30 (-5.9589, 18.3076) -> (-4.1691, 15.2076) projected
  line L31 (-4.1691, 15.2076) -> (-5.9589, 12.1076) projected
  line L32 (-5.9589, 12.1076) -> (-9.5385, 12.1076) projected
  line L33 (-9.5385, 12.1076) -> (-11.3283, 15.2076) projected
  line L34 (-11.3283, 15.2076) -> (-9.5385, 18.3076) projected
  line L35 (-9.5385, 18.3076) -> (-5.9589, 18.3076) projected
  circle A8 centre (3.2428, 61.8766) radius 4 projected
  circle A9 centre (28.1299, -55.2081) radius 4 projected
  circle A10 centre (-3.2428, -61.8766) radius 4 projected
  circle A11 centre (-33.7467, -51.9653) radius 4 projected
  circle A12 centre (33.7467, 51.9653) radius 4 projected
  circle A13 centre (-28.1299, 55.2081) radius 4 projected
  line L36 (-7.7487, 15.2076) -> (-5.064, 13.6576)
  line L37 (-4.1691, 15.2076) -> (-5.9589, 12.1076) projected
  line L38 (-7.7487, 15.2076) -> (-4.7176, 13.4576)
  line L39 (-7.7487, 15.2076) -> (-10.4334, 16.7576)
  line L40 (-11.3283, 15.2076) -> (-9.5385, 18.3076) projected
  line L41 (-5.728, 11.7076) -> (-9.7694, 11.7076)
  line L42 (-9.7694, 11.7076) -> (-11.7901, 15.2076)
  line L43 (-11.7901, 15.2076) -> (-9.7694, 18.7076)
  line L44 (-9.7694, 18.7076) -> (-5.728, 18.7076)
  line L45 (-5.728, 18.7076) -> (-3.7072, 15.2076)
  line L46 (-3.7072, 15.2076) -> (-5.728, 11.7076)
  line L47 (-13.0031, 0.8933) -> (-15.0238, -2.6067)
  line L48 (-15.0238, 4.3933) -> (-13.0031, 0.8933)
  line L49 (-19.0653, 4.3933) -> (-15.0238, 4.3933)
  line L50 (-21.086, 0.8933) -> (-19.0653, 4.3933)
  line L51 (-19.0653, -2.6067) -> (-21.086, 0.8933)
  line L52 (-15.0238, -2.6067) -> (-19.0653, -2.6067)
  line L53 (-7.2751, -10.8144) -> (-5.2544, -14.3144)
  line L54 (-11.3166, -10.8144) -> (-7.2751, -10.8144)
  line L55 (-13.3373, -14.3144) -> (-11.3166, -10.8144)
  line L56 (-11.3166, -17.8144) -> (-13.3373, -14.3144)
  line L57 (-7.2751, -17.8144) -> (-11.3166, -17.8144)
  line L58 (-5.2544, -14.3144) -> (-7.2751, -17.8144)
  line L59 (5.728, -11.7076) -> (9.7694, -11.7076)
  line L60 (3.7072, -15.2076) -> (5.728, -11.7076)
  line L61 (5.728, -18.7076) -> (3.7072, -15.2076)
  line L62 (9.7694, -18.7076) -> (5.728, -18.7076)
  line L63 (11.7901, -15.2076) -> (9.7694, -18.7076)
  line L64 (9.7694, -11.7076) -> (11.7901, -15.2076)
  line L65 (13.0031, -0.8933) -> (15.0238, 2.6067)
  line L66 (15.0238, -4.3933) -> (13.0031, -0.8933)
  line L67 (19.0653, -4.3933) -> (15.0238, -4.3933)
  line L68 (21.086, -0.8933) -> (19.0653, -4.3933)
  line L69 (19.0653, 2.6067) -> (21.086, -0.8933)
  line L70 (15.0238, 2.6067) -> (19.0653, 2.6067)
  line L71 (7.2751, 10.8144) -> (5.2544, 14.3144)
  line L72 (11.3166, 10.8144) -> (7.2751, 10.8144)
  line L73 (13.3373, 14.3144) -> (11.3166, 10.8144)
  line L74 (11.3166, 17.8144) -> (13.3373, 14.3144)
  line L75 (7.2751, 17.8144) -> (11.3166, 17.8144)
  line L76 (5.2544, 14.3144) -> (7.2751, 17.8144)
  point P0 (1.3155, -25.1014)
  point P1 (-14.0135, 2.6433)
  point P2 (-9.2959, -10.8144)
  point P3 (4.7176, -13.4576)
  point P4 (14.0135, -2.6433)
  point P5 (9.2959, 10.8144)
  dimension "d92" = 3.5
  dimension "d95" = 360
  constraints: 78 end point, 3 midpoint, 1 coincident, 1 point on line, 92 other
  measures "d92" distance of L36.start L38.end
extrude "Extrusion23" cut sketch "Sketch21" against normal up to surface (10.4 mm away) contours A0 | A1 | A2 | A3 | A4 | A5 L36 L39 | A5 L39 L34 L35 L30 L31 L36 | L39 L36 A5 | A5 L36 L31 L32 L33 L34 L39 | L0 L1 L2 L3 L4 L5 | L6 L7 L8 L9 L10 L11 | L12 L13 L14 L15 L16 L17 | L18 L19 L20 L21 L22 L23 | L24 L25 L26 L27 L28 L29 | L41 L42 L43 L44 L45 L46 | L47 L52 L51 L50 L49 L48 | L53 L58 L57 L56 L55 L54 | L59 L64 L63 L62 L61 L60 | L65 L70 L69 L68 L67 L66 | L71 L76 L75 L74 L73 L72
sketch "Sketch22" plane through (-1.3155, 25.1014, 42) normal (0, 0, 1) x (1, 0, 0)
  line L0 (5.728, -11.7076) -> (9.7694, -11.7076) projected
  line L1 (9.7694, -11.7076) -> (11.7901, -15.2076) projected
  line L2 (11.7901, -15.2076) -> (9.7694, -18.7076) projected
  line L3 (9.7694, -18.7076) -> (5.728, -18.7076) projected
  line L4 (5.728, -18.7076) -> (3.7072, -15.2076) projected
  line L5 (3.7072, -15.2076) -> (5.728, -11.7076) projected
  line L6 (5.2544, 14.3144) -> (7.2751, 17.8144) projected
  line L7 (7.2751, 17.8144) -> (11.3166, 17.8144) projected
  line L8 (11.3166, 17.8144) -> (13.3373, 14.3144) projected
  line L9 (13.3373, 14.3144) -> (11.3166, 10.8144) projected
  line L10 (11.3166, 10.8144) -> (7.2751, 10.8144) projected
  line L11 (7.2751, 10.8144) -> (5.2544, 14.3144) projected
  line L12 (-13.0031, 0.8933) -> (-15.0238, -2.6067) projected
  line L13 (-15.0238, -2.6067) -> (-19.0653, -2.6067) projected
  line L14 (-19.0653, -2.6067) -> (-21.086, 0.8933) projected
  line L15 (-21.086, 0.8933) -> (-19.0653, 4.3933) projected
  line L16 (-19.0653, 4.3933) -> (-15.0238, 4.3933) projected
  line L17 (-15.0238, 4.3933) -> (-13.0031, 0.8933) projected
  line L18 (-5.2544, -14.3144) -> (-7.2751, -17.8144) projected
  line L19 (-7.2751, -17.8144) -> (-11.3166, -17.8144) projected
  line L20 (-11.3166, -17.8144) -> (-13.3373, -14.3144) projected
  line L21 (-13.3373, -14.3144) -> (-11.3166, -10.8144) projected
  line L22 (-11.3166, -10.8144) -> (-7.2751, -10.8144) projected
  line L23 (-7.2751, -10.8144) -> (-5.2544, -14.3144) projected
  line L24 (13.0031, -0.8933) -> (15.0238, 2.6067) projected
  line L25 (15.0238, 2.6067) -> (19.0653, 2.6067) projected
  line L26 (19.0653, 2.6067) -> (21.086, -0.8933) projected
  line L27 (21.086, -0.8933) -> (19.0653, -4.3933) projected
  line L28 (19.0653, -4.3933) -> (15.0238, -4.3933) projected
  line L29 (15.0238, -4.3933) -> (13.0031, -0.8933) projected
  line L30 (-9.7694, 11.7076) -> (-11.7901, 15.2076) projected
  line L31 (-11.7901, 15.2076) -> (-9.7694, 18.7076) projected
  line L32 (-9.7694, 18.7076) -> (-5.728, 18.7076) projected
  line L33 (-5.728, 18.7076) -> (-3.7072, 15.2076) projected
  line L34 (-3.7072, 15.2076) -> (-5.728, 11.7076) projected
  line L35 (-5.728, 11.7076) -> (-9.7694, 11.7076) projected
  circle A0 centre (0, 0) radius 70 projected
  circle A1 centre (0, 0) radius 8 projected
  circle A2 centre (3.2428, 61.8766) radius 4 projected
  circle A3 centre (28.1299, -55.2081) radius 4 projected
  circle A4 centre (-3.2428, -61.8766) radius 4 projected
  circle A5 centre (-33.7467, -51.9653) radius 4 projected
  circle A6 centre (33.7467, 51.9653) radius 4 projected
  circle A7 centre (-28.1299, 55.2081) radius 4 projected
  circle A8 centre (-7.7487, 15.2076) radius 2 projected
  circle A9 centre (-7.7487, 15.2076) radius 4.1
  circle A10 centre (-17.0446, 0.8933) radius 4.1
  circle A11 centre (-9.2959, -14.3144) radius 4.1
  circle A12 centre (7.7487, -15.2076) radius 4.1
  circle A13 centre (17.0446, -0.8933) radius 4.1
  circle A14 centre (9.2959, 14.3144) radius 4.1
  point P0 (1.3155, -25.1014)
  dimension "d99" = 8.2
  dimension "d102" = 360
  constraints: 6 centre point, 1 coincident, 13 other
  measures "d99" diameter of A9
extrude "Extrusion24" cut sketch "Sketch22" against normal blind 5.4 contours L0 L1 L2 L3 L4 L5 | L6 L7 L8 L9 L10 L11 | L12 L13 L14 L15 L16 L17 | L18 L19 L20 L21 L22 L23 | L24 L25 L26 L27 L28 L29 | L30 L31 L32 L33 L34 L35 | A8 | A9 | A10 | A11 | A12 | A13 | A14
fillet "Fillet3" radius 0.3 7 edges at (-9.3155, 25.1014, 42) (11.629, 24.2082, 42) (2.3332, 9.8938, 42) (-14.7114, 10.7871, 42) (-22.4601, 25.9947, 42) (-13.1642, 40.3091, 42) (3.8804, 39.4158, 42)
fillet "Fillet4" radius 0.3 8 edges at (28.4312, 77.0667, 42) (-2.0727, 86.978, 42) (-33.4455, 80.3096, 42) (22.8144, -30.1067, 42) (-8.5583, -36.7752, 42) (-39.0622, -26.8639, 42) (-71.3155, 25.1014, 27) (-71.3155, 25.1014, 42)
body "Solid1"
